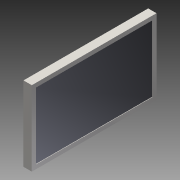
# Autodesk Inventor part: Television
Saved by Autodesk Inventor 2015 SP1 (Build 190203100, 203)
## iProperties
Created: 2016-02-03
Part Number: Television
Material: Generic
Document SubType Name: Modeling
Designer: guillemd
Mass: 6803.89 g
Surface Area: 8263.21 cm^2
Volume: 16963.9 cm^3
Density: 0.384443 g/cm^3
Appearance: Titanium
Author: guillemd
Autodesk Inventor part; units mm, degrees
ref_plane "YZ Plane" through (0, 0, 0) normal (1, 0, 0) x (0, 1, 0)
ref_plane "XZ Plane" through (0, 0, 0) normal (0, 1, 0) x (-1, 0, 0)
ref_plane "XY Plane" through (0, 0, 0) normal (0, 0, 1) x (1, 0, 0)
sketch "Sketch1" plane through (0, 0, 0) normal (1, 0, 0) x (0, 1, 0)
  line L0 (228.6, 381) -> (-228.6, 381)
  line L1 (-228.6, 381) -> (-228.6, -381)
  line L2 (-228.6, -381) -> (228.6, -381)
  line L3 (228.6, -381) -> (228.6, 381)
  point P0 (0, 0)
  point P1 (228.6, 0)
  point P2 (0, -381)
  dimension "d0" = 762
  dimension "d1" = 457.2
  constraints: 8 end point, 2 midpoint, 2 parallel, 1 horizontal, 1 horizontal alignment, 1 perpendicular, 1 vertical alignment
  measures "d0" distance of L2.end L0.start
  measures "d1" distance of L1.end L2.end
extrude "Extrusion1" add sketch "Sketch1" along normal blind 50.8
sketch "Sketch2" plane through (50.8, 0, 0) normal (1, 0, 0) x (0, 0, -1)
  line L0 (381, 228.6) -> (-381, 228.6) projected
  line L1 (-381, 228.6) -> (-381, -228.6) projected
  line L2 (-381, -228.6) -> (381, -228.6) projected
  line L3 (381, -228.6) -> (381, 228.6) projected
  line L4 (-355.6, 203.2) -> (355.6, 203.2)
  line L5 (355.6, 203.2) -> (355.6, -203.2)
  line L6 (355.6, -203.2) -> (-355.6, -203.2)
  line L7 (-355.6, -203.2) -> (-355.6, 203.2)
  point P0 (0, 0)
  dimension "d4" = 25.4
  constraints: 8 end point, 3 other
  measures "d4" distance between parallel lines of L0 L4
extrude "Extrusion2" cut sketch "Sketch2" against normal blind 2.54 contours L4 L5 L6 L7
body "Solid1"
